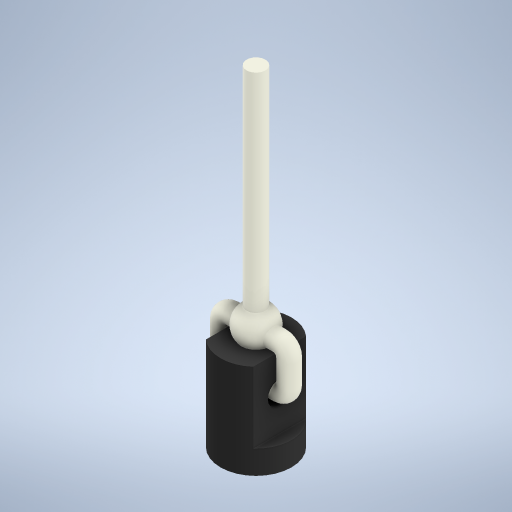
# Autodesk Inventor part: dummy_anchor_end_3.0mm_w_string
Saved by Autodesk Inventor 2024.3 (Build 283343000, 343)
## iProperties
Created: 2024-06-07
Part Number: dummy_anchor_end_3.0mm_w_string
Material: 일반
Document SubType Name: Modeling
Designer: Gihyeok Na
Density: 1 g/cm^3
Appearance: 기본값
Author: Gihyeok Na
Autodesk Inventor part; units mm, degrees
ref_plane "YZ Plane" through (0, 0, 0) normal (1, 0, 0) x (0, 1, 0)
ref_plane "XZ Plane" through (0, 0, 0) normal (0, 1, 0) x (-1, 0, 0)
sketch "스케치2" plane through (0, 0, 0) normal (0, 1, 0) x (-1, 0, 0)
  circle A0 centre (0, 0) radius 1.5
  circle A1 centre (0, 0) radius 0.9
  dimension "d0" = 3
  dimension "d6" = 1.8
  constraints: 2 centre point, 2 coincident
  measures "d0" diameter of A0
  measures "d6" diameter of A1
extrude "돌출1" add sketch "스케치2" along normal blind 1
sketch "스케치4" plane through (0, 1, 0) normal (0, 1, 0) x (1, 0, 0)
  line L0 (1, -3.1) -> (-1, -3.1)
  line L1 (-1, -3.1) -> (-1, 3.1)
  line L2 (-1, 3.1) -> (1, 3.1)
  line L3 (1, 3.1) -> (1, -3.1)
  line L4 (1, -3.1) -> (-1, 3.1) construction
  line L5 (-1, -3.1) -> (1, 3.1) construction
  circle A0 centre (0, 0) radius 1.5 projected
  point P0 (1, 1.118034)
  point P1 (-1, 1.118034)
  point P2 (-1, -1.118034)
  point P3 (1, -1.118034)
  dimension "d7" = 2
  constraints: 12 end point, 2 midpoint, 2 parallel, 1 horizontal, 1 perpendicular
  measures "d7" distance of L1.end L2.end
extrude "돌출5" add sketch "스케치4" along normal blind 3 contours A0 L1 L3
sketch "스케치6" plane through (1, 1, 1.118034) normal (1, 0, 0) x (0, 0, -1)
  circle A0 centre (1.118034, 1.5) radius 0.5
  line L0 (0, 3) -> (2.236068, 3)
  point P0 (1.118034, -1)
  dimension "d22" = 1
  dimension "d23" = 1.5
  constraints: 1 centre point
  measures "d22" diameter of A0
  measures "d23" distance from line of L0 A0.centre
extrude "돌출6" cut sketch "스케치6" along normal through all both and the other way through all
sketch "Sketch7" plane through (0, 4, 0) normal (0, 1, 0) x (1, 0, 0)
  circle A0 centre (0, 0) radius 0.4
  dimension "d26" = 0.8
  constraints: 1 centre point, 1 coincident
  measures "d26" diameter of A0
extrude "Extrusion7" add sketch "Sketch7" along normal blind 10
sketch "Sketch8" plane through (0, 0, 0) normal (0, 0, 1) x (1, 0, 0)
  line L0 (0.264968, 4.4) -> (-1, 4.4)
  line L1 (-1.4, 4) -> (-1.4, 3)
  line L2 (-1, 2.6) -> (0.264968, 2.6)
  line L3 (1, 4) -> (-1, 4)
  line L4 (0.264968, 4.4) -> (1, 4.4)
  line L5 (1.4, 4) -> (1.4, 3)
  line L6 (1, 2.6) -> (0.264968, 2.6)
  line L7 (1, 1) -> (1, 4)
  line L8 (-1, 1) -> (-1, 4)
  arc A0 (-1, 4.4) -> (-1.4, 4) centre (-1, 4) ccw
  arc A1 (1.4, 4) -> (1, 4.4) centre (1, 4) ccw
  line L9 (-1, 3) -> (1, 3)
  arc A2 (-1.4, 3) -> (-1, 2.6) centre (-1, 3) ccw
  arc A3 (1, 2.6) -> (1.4, 3) centre (1, 3) ccw
  point P0 (0, 0)
  dimension "d29" = 0.4
  dimension "d30" = 1.4
  dimension "d32" = 0.4
  dimension "d33" = 0.4
  constraints: 12 end point, 8 point on circle, 6 point on line, 4 centre point, 2 coincident, 2 horizontal, 2 perpendicular, 1 collinear, 1 parallel
  measures "d29" distance between parallel lines of L0 L3
  measures "d30" distance between parallel lines of L2 L3
  measures "d32" distance from line of L3.end L1
  measures "d33" distance between parallel lines of L5 L7
sketch "Sketch9" plane through (0, 0, 0) normal (1, 0, 0) x (0, 1, 0)
  circle A0 centre (4.4, 0) radius 0.39
  line L0 (14, -0.4) -> (14, 0.4) projected
  line L1 (4, 0.4) -> (4, -0.4) projected
  point P0 (0, 0)
  dimension "d34" = 0.78
  constraints: 1 centre point, 1 coincident
  measures "d34" diameter of A0
sweep "Sweep1" add profiles "Sketch9" path "Sketch8" path curves L0 A0 L1 A2 L2 L6 A3 L5 A1 L4
ref_plane "Work Plane2" through (0, 4.5, 0) normal (0, 1, 0) x (1, 0, 0)
sketch "Sketch11" plane through (0, 4.5, 0) normal (0, 1, 0) x (1, 0, 0)
  circle A0 centre (0, 0) radius 0.9 projected
  circle A1 centre (0, 0) radius 0.8
  line L0 (0, -0.8) -> (0, 0.8)
  dimension "d40" = 1.6
  constraints: 2 end point, 2 point on circle, 1 centre point, 1 coincident, 1 vertical
  measures "d40" diameter of A1
sketch "Sketch11 outline for Revolution2" plane through (0, 4.5, 0) normal (0, 1, 0) x (1, 0, 0)
  line L0 (0, 0.8) -> (0, -0.8)
  arc A0 (0, -0.8) -> (0, 0.8) centre (0, 0) ccw
revolve "Revolution2" add sketch "Sketch11 outline for Revolution2" angle 360 about axis through (0, 4.5, 0.8) along (0, 0, -1)
